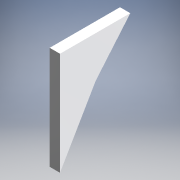
# Autodesk Inventor part: 앞판바깥막이
Saved by Autodesk Inventor 2017 (Build 210142000, 142)
## iProperties
Part Number: 앞판바깥막이
Material: 알루미늄 6061
Document SubType Name: Modeling
Designer: minom
Mass: 10.4495 g
Surface Area: 22.7233 cm^2
Volume: 3.87019 cm^3
Density: 2.7 g/cm^3
Appearance: 알루미늄 - 평지
Author: minom
Autodesk Inventor part; units mm, degrees
ref_plane "YZ Plane" through (0, 0, 0) normal (1, 0, 0) x (0, 1, 0)
ref_plane "XZ Plane" through (0, 0, 0) normal (0, 1, 0) x (-1, 0, 0)
ref_plane "XY Plane" through (0, 0, 0) normal (0, 0, 1) x (1, 0, 0)
sketch "스케치1" plane through (0, 0, 0) normal (1, 0, 0) x (0, 1, 0)
  line L0 (0, 0) -> (0, 30)
  line L1 (0, 0) -> (30, 0) construction
  line L2 (0, 30) -> (0, 50)
  line L3 (0, 50) -> (31.958, 50)
  line L4 (0, 0) -> (17.3205, 30)
  line L5 (0, 0) -> (34.641, 0) construction
  line L6 (17.3205, 30) -> (32.724, 48.3572)
  arc A0 (32.724, 48.3572) -> (31.958, 50) centre (31.958, 49) ccw
  point P0 (34.1025, 50)
  dimension "d0" = 30
  dimension "d1" = 90
  dimension "d2" = 20
  dimension "d3" = 60
  dimension "d4" = 170
  dimension "d7" = 1
  constraints: 14 end point, 3 point on line, 2 equal length, 2 horizontal, 2 point on circle, 2 tangent, 1 centre point, 1 perpendicular, 1 vertical
  measures "d0" distance of L0.start L0.end
  measures "d1" angle of L1 L0
  measures "d2" distance of L0.end L2.end
  measures "d3" angle of L5 L4
  measures "d4" angle of L4 L6
  measures "d7" radius of A0
extrude "돌출1" add sketch "스케치1" along normal blind 5
